planet holder (Autodesk Fusion 360 design; units mm, degrees)
part number: 2026-06-12-03-12-57-435
Autodesk Fusion 360 part; units mm, degrees
note: some values were not read from the file. Set by a fixed rule: which sketch regions a step uses.
sketch "Sketch1" plane through (0, 0, 0) normal (0, 1, 0) x (1, 0, 0)
  circle A0 centre (0, 0) radius 15.145
  circle A1 centre (0, 17.145) radius 4
  circle A2 centre (-14.848, -8.5725) radius 4
  circle A3 centre (14.848, -8.5725) radius 4
  circle A4 centre (0, 0) radius 9
  circle A5 centre (0, 17) radius 6
  circle A6 centre (-14.7224, -8.5) radius 6
  circle A7 centre (14.7224, -8.5) radius 6
  dimension "d3" = 30.29
  dimension "d4" = 8
  dimension "d7" = 18
  dimension "d9" = 360
  constraint concentric A0 A4
  measures "d3" diameter of A0
  measures "d4" diameter of A1
  measures "d7" diameter of A4
extrude "Extrude1" add sketch "Sketch1" along normal blind 3 contours A0 A5 A6 A7 | A0 A1 A5 | A0 A1 A5 | A0 A3 A7 | A0 A3 A7 | A0 A2 A6 | A0 A2 A6
